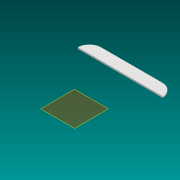
# Autodesk Inventor part: 导轨
Saved by Autodesk Inventor 2021 (Build 250183000, 183)
## iProperties
Created: 2025-04-17
Part Number: 导轨
Material: 常规
Document SubType Name: Modeling
Designer: 86155
Density: 1 g/cm^3
Appearance: 默认
Author: 86155
Autodesk Inventor part; units mm, degrees
ref_plane "YZ Plane" through (0, 0, 0) normal (1, 0, 0) x (0, 1, 0)
ref_plane "XZ Plane" through (0, 0, 0) normal (0, 1, 0) x (-1, 0, 0)
ref_plane "XY Plane" through (0, 0, 0) normal (0, 0, 1) x (1, 0, 0)
ref_plane "工作平面1" through (0, 0, 0) normal (0, -1, 0) x (1, 0, 0)
sketch "草图2" plane through (0, 0, 0) normal (0, -1, 0) x (1, 0, 0)
  line L0 (13.9089, -43.2782) -> (-26.0911, -43.2782) projected
  arc A0 (13.9089, -43.2782) -> (21.4089, -35.7782) centre (13.9089, -35.7782) ccw projected
  line L1 (-33.5911, -35.7782) -> (21.4089, -35.7782) projected
  arc A1 (-33.5911, -35.7782) -> (-26.0911, -43.2782) centre (-26.0911, -35.7782) ccw projected
  point P0 (0, 0)
extrude "拉伸2" add sketch "草图2" along normal blind 2
ref_plane "工作平面2" through (-1.2405, 0, -40.1772) normal (0, -1, 0) x (1, 0, 0)
sketch "草图3" plane through (0, -2, 0) normal (0, -1, 0) x (1, 0, 0)
  line L0 (-21.0911, -35.7782) -> (8.9089, -35.7782)
  line L1 (8.9089, -35.7782) -> (8.9089, -43.7782)
  line L2 (8.9089, -43.7782) -> (-21.0911, -43.7782)
  line L3 (21.4089, -35.7782) -> (-33.5911, -35.7782) projected
  line L4 (-21.0911, -38.7782) -> (-19.5911, -38.7782)
  line L5 (-19.5911, -38.7782) -> (-19.5911, -39.7782)
  line L6 (-19.5911, -39.7782) -> (-21.0911, -39.7782)
  line L7 (-21.0911, -43.7782) -> (-21.0911, -39.7782)
  line L8 (-21.0911, -38.7782) -> (-21.0911, -35.7782)
  line L9 (8.9089, -39.7782) -> (7.4089, -39.7782)
  line L10 (7.4089, -39.7782) -> (7.4089, -38.7782)
  line L11 (7.4089, -38.7782) -> (8.9089, -38.7782)
  line L12 (8.9089, -38.7782) -> (8.9089, -39.7782)
  point P0 (0, 0)
  dimension "d7" = 8
  dimension "d8" = 1
  dimension "d9" = 3
  dimension "d10" = 1.5
  dimension "d11" = 1.5
  constraints: 24 end point, 6 parallel, 3 horizontal, 3 perpendicular, 1 collinear, 1 midpoint
  measures "d7" distance between parallel lines of L2 L0
  measures "d8" distance between parallel lines of L6 L4
  measures "d9" distance between parallel lines of L0 L4
  measures "d10" distance between parallel lines of L8 L5
  measures "d11" distance of L10.end L11.end
extrude "拉伸3" add sketch "草图3" along normal blind 345 contours L0 L1 L11 L10 L9 L2 L7 L6 L5 L4 L8
ref_plane "工作平面3" through (0, -174.5, 0) normal (0, -1, 0) x (1, 0, 0)
mirror "镜像1" about plane through (0, -174.5, 0) normal (0, -1, 0) of "拉伸2"
